Autodesk Fusion 360 part; units mm, degrees
(part 3 of 5)
sketch "スケッチ1 (2)" plane through (0, 0, 0) normal (0, 0, 1) x (1, 0, 0) in component "CasePlateExtended"
  spline S0 degree 3 poles (160.1864, -37.956) (159.9114, -37.956) (159.6865, -37.7311) (159.6865, -37.456) knots 0 0 0 0 1 1 1 1
  line L0 (159.6865, -37.456) -> (159.6865, -33.7563)
  spline S1 degree 3 poles (159.6865, -33.7563) (159.6865, -33.4812) (159.4615, -33.2562) (159.1863, -33.2562) knots 2 2 2 2 3 3 3 3
  line L1 (159.1863, -33.2562) -> (158.7622, -33.2562)
  spline S2 degree 3 poles (158.7622, -33.2562) (158.4869, -33.2562) (158.2619, -33.4812) (158.2619, -33.7563) knots 4 4 4 4 5 5 5 5
  line L2 (158.2619, -33.7563) -> (158.2619, -37.456)
  spline S3 degree 3 poles (158.2619, -37.456) (158.2619, -37.7311) (158.037, -37.956) (157.7621, -37.956) knots 6 6 6 6 7 7 7 7
  line L3 (157.7621, -37.956) -> (157.0372, -37.956)
  spline S4 degree 3 poles (157.0372, -37.956) (156.7619, -37.956) (156.537, -38.1743) (156.537, -38.7079) (156.312, -38.9262) (156.0371, -38.9262) knots 8 8 8 8 9 9 10 10 10 10
  line L4 (156.0371, -38.9262) -> (153.3871, -38.9262)
  spline S5 degree 3 poles (153.3871, -38.9262) (153.1119, -38.9262) (152.8869, -38.7079) (152.8869, -38.1743) (152.6619, -37.956) (152.387, -37.956) knots 11 11 11 11 12 12 13 13 13 13
  line L5 (152.387, -37.956) -> (143.5186, -37.956)
  spline S6 degree 3 poles (143.5186, -37.956) (143.2437, -37.956) (143.0188, -37.7311) (143.0188, -37.456) knots 14 14 14 14 15 15 15 15
  line L6 (143.0188, -37.456) -> (143.0188, -24.4562)
  spline S7 degree 3 poles (143.0188, -24.4562) (143.0188, -24.1811) (143.2437, -23.9562) (143.5186, -23.9562) knots 16 16 16 16 17 17 17 17
  line L7 (143.5186, -23.9562) -> (156.5184, -23.9562)
  spline S8 degree 3 poles (156.5184, -23.9562) (156.7936, -23.9562) (157.0186, -24.1744) (157.0186, -24.7077) (157.2436, -24.926) (157.5185, -24.926) knots 18 18 18 18 19 19 20 20 20 20
  line L8 (157.5185, -24.926) -> (157.7621, -24.926)
  spline S9 degree 3 poles (157.7621, -24.926) (158.037, -24.926) (158.2619, -25.1509) (158.2619, -25.426) knots 21 21 21 21 22 22 22 22
  line L9 (158.2619, -25.426) -> (158.2619, -28.1559)
  spline S10 degree 3 poles (158.2619, -28.1559) (158.2619, -28.431) (158.4869, -28.656) (158.7622, -28.656) knots 23 23 23 23 24 24 24 24
  line L10 (158.7622, -28.656) -> (159.1863, -28.656)
  spline S11 degree 3 poles (159.1863, -28.656) (159.4615, -28.656) (159.6865, -28.431) (159.6865, -28.1559) knots 25 25 25 25 26 26 26 26
  line L11 (159.6865, -28.1559) -> (159.6865, -24.4562)
  spline S12 degree 3 poles (159.6865, -24.4562) (159.6865, -24.1811) (159.9114, -23.9562) (160.1864, -23.9562) knots 27 27 27 27 28 28 28 28
  line L12 (160.1864, -23.9562) -> (182.7114, -23.9562)
  spline S13 degree 3 poles (182.7114, -23.9562) (182.9867, -23.9562) (183.2117, -24.1811) (183.2117, -24.4562) knots 29 29 29 29 30 30 30 30
  line L13 (183.2117, -24.4562) -> (183.2117, -37.456)
  spline S14 degree 3 poles (183.2117, -37.456) (183.2117, -37.7311) (182.9867, -37.956) (182.7114, -37.956) knots 31 31 31 31 32 32 32 32
  line L14 (182.7114, -37.956) -> (180.9861, -37.956)
  spline S15 degree 3 poles (180.9861, -37.956) (180.7109, -37.956) (180.4859, -38.1743) (180.4859, -38.7079) (180.261, -38.9262) (179.986, -38.9262) knots 33 33 33 33 34 34 35 35 35 35
  line L15 (179.986, -38.9262) -> (177.3371, -38.9262)
  spline S16 degree 3 poles (177.3371, -38.9262) (177.0618, -38.9262) (176.8369, -38.7079) (176.8369, -38.1743) (176.6119, -37.956) (176.337, -37.956) knots 36 36 36 36 37 37 38 38 38 38
  line L16 (176.337, -37.956) -> (160.1864, -37.956)
  spline S17 degree 3 poles (114.4437, -5.4062) (114.4437, -5.1311) (114.6687, -4.9062) (114.9436, -4.9062) knots 0 0 0 0 1 1 1 1
  line L17 (114.9436, -4.9062) -> (127.9434, -4.9062)
  spline S18 degree 3 poles (127.9434, -4.9062) (128.2186, -4.9062) (128.4436, -5.1311) (128.4436, -5.4062) knots 2 2 2 2 3 3 3 3
  line L18 (128.4436, -5.4062) -> (128.4436, -18.406)
  spline S19 degree 3 poles (128.4436, -18.406) (128.4436, -18.681) (128.2186, -18.906) (127.9434, -18.906) knots 4 4 4 4 5 5 5 5
  line L19 (127.9434, -18.906) -> (114.9436, -18.906)
  spline S20 degree 3 poles (114.9436, -18.906) (114.6687, -18.906) (114.4437, -18.681) (114.4437, -18.406) knots 6 6 6 6 7 7 7 7
  line L20 (114.4437, -18.406) -> (114.4437, -5.4062)
  spline S21 degree 3 poles (110.1804, 0.144) (109.9055, 0.144) (109.6805, 0.369) (109.6805, 0.6441) knots 0 0 0 0 1 1 1 1
  line L21 (109.6805, 0.6441) -> (109.6805, 13.6438)
  spline S22 degree 3 poles (109.6805, 13.6438) (109.6805, 13.9189) (109.9055, 14.1438) (110.1804, 14.1438) knots 2 2 2 2 3 3 3 3
  line L22 (110.1804, 14.1438) -> (123.1805, 14.1438)
  spline S23 degree 3 poles (123.1805, 14.1438) (123.4558, 14.1438) (123.6807, 13.9189) (123.6807, 13.6438) knots 4 4 4 4 5 5 5 5
  line L23 (123.6807, 13.6438) -> (123.6807, 0.6441)
  spline S24 degree 3 poles (123.6807, 0.6441) (123.6807, 0.369) (123.4558, 0.144) (123.1805, 0.144) knots 6 6 6 6 7 7 7 7
  line L24 (123.1805, 0.144) -> (110.1804, 0.144)
  line L25 (198.3818, 67.532) -> (-198.3818, 67.532)
  spline S25 degree 3 poles (-198.3818, 67.532) (-199.7568, 67.532) (-200.8816, 66.407) (-200.8816, 65.0321) knots 1 1 1 1 2 2 2 2
  line L26 (-200.8816, 65.0321) -> (-200.8816, -65.0319)
  spline S26 degree 3 poles (-200.8816, -65.0319) (-200.8816, -66.4072) (-199.7568, -67.532) (-198.3818, -67.532) knots 3 3 3 3 4 4 4 4
  line L27 (-198.3818, -67.532) -> (198.3818, -67.532)
  spline S27 degree 3 poles (198.3818, -67.532) (199.7564, -67.532) (200.8816, -66.4072) (200.8816, -65.0319) knots 5 5 5 5 6 6 6 6
  line L28 (200.8816, -65.0319) -> (200.8816, 65.0321)
  spline S28 degree 3 poles (200.8816, 65.0321) (200.8816, 66.407) (199.7564, 67.532) (198.3818, 67.532) knots 7 7 7 7 8 8 8 8
  spline S29 degree 3 poles (91.1304, 0.144) (90.8555, 0.144) (90.6305, 0.369) (90.6305, 0.6441) knots 0 0 0 0 1 1 1 1
  line L29 (90.6305, 0.6441) -> (90.6305, 13.6438)
  spline S30 degree 3 poles (90.6305, 13.6438) (90.6305, 13.9189) (90.8555, 14.1438) (91.1304, 14.1438) knots 2 2 2 2 3 3 3 3
  line L30 (91.1304, 14.1438) -> (104.1305, 14.1438)
  spline S31 degree 3 poles (104.1305, 14.1438) (104.4058, 14.1438) (104.6307, 13.9189) (104.6307, 13.6438) knots 4 4 4 4 5 5 5 5
  line L31 (104.6307, 13.6438) -> (104.6307, 0.6441)
  spline S32 degree 3 poles (104.6307, 0.6441) (104.6307, 0.369) (104.4058, 0.144) (104.1305, 0.144) knots 6 6 6 6 7 7 7 7
  line L32 (104.1305, 0.144) -> (91.1304, 0.144)
  spline S33 degree 3 poles (157.3056, 56.506) (157.3056, 56.7811) (157.5305, 57.006) (157.8055, 57.006) knots 0 0 0 0 1 1 1 1
  line L33 (157.8055, 57.006) -> (170.8055, 57.006)
  spline S34 degree 3 poles (170.8055, 57.006) (171.0808, 57.006) (171.3058, 56.7811) (171.3058, 56.506) knots 2 2 2 2 3 3 3 3
  line L34 (171.3058, 56.506) -> (171.3058, 43.5059)
  spline S35 degree 3 poles (171.3058, 43.5059) (171.3058, 43.2308) (171.0808, 43.0058) (170.8055, 43.0058) knots 4 4 4 4 5 5 5 5
  line L35 (170.8055, 43.0058) -> (157.8055, 43.0058)
  spline S36 degree 3 poles (157.8055, 43.0058) (157.5305, 43.0058) (157.3056, 43.2308) (157.3056, 43.5059) knots 6 6 6 6 7 7 7 7
  line L36 (157.3056, 43.5059) -> (157.3056, 56.506)
  spline S37 degree 3 poles (129.2304, 0.144) (128.9555, 0.144) (128.7306, 0.369) (128.7306, 0.6441) knots 0 0 0 0 1 1 1 1
  line L37 (128.7306, 0.6441) -> (128.7306, 13.6438)
  spline S38 degree 3 poles (128.7306, 13.6438) (128.7306, 13.9189) (128.9555, 14.1438) (129.2304, 14.1438) knots 2 2 2 2 3 3 3 3
  line L38 (129.2304, 14.1438) -> (142.2305, 14.1438)
  spline S39 degree 3 poles (142.2305, 14.1438) (142.5058, 14.1438) (142.7307, 13.9189) (142.7307, 13.6438) knots 4 4 4 4 5 5 5 5
  line L39 (142.7307, 13.6438) -> (142.7307, 0.6441)
  spline S40 degree 3 poles (142.7307, 0.6441) (142.7307, 0.369) (142.5058, 0.144) (142.2305, 0.144) knots 6 6 6 6 7 7 7 7
  line L40 (142.2305, 0.144) -> (129.2304, 0.144)
  spline S41 degree 3 poles (119.2056, 32.6938) (119.2056, 32.9689) (119.4305, 33.1939) (119.7054, 33.1939) knots 0 0 0 0 1 1 1 1
  line L41 (119.7054, 33.1939) -> (132.7055, 33.1939)
  spline S42 degree 3 poles (132.7055, 33.1939) (132.9808, 33.1939) (133.2057, 32.9689) (133.2057, 32.6938) knots 2 2 2 2 3 3 3 3
  line L42 (133.2057, 32.6938) -> (133.2057, 19.6941)
  spline S43 degree 3 poles (133.2057, 19.6941) (133.2057, 19.419) (132.9808, 19.194) (132.7055, 19.194) knots 4 4 4 4 5 5 5 5
  line L43 (132.7055, 19.194) -> (119.7054, 19.194)
  spline S44 degree 3 poles (119.7054, 19.194) (119.4305, 19.194) (119.2056, 19.419) (119.2056, 19.6941) knots 6 6 6 6 7 7 7 7
  line L44 (119.2056, 19.6941) -> (119.2056, 32.6938)
  spline S45 degree 3 poles (138.2556, 56.506) (138.2556, 56.7811) (138.4805, 57.006) (138.7554, 57.006) knots 0 0 0 0 1 1 1 1
  line L45 (138.7554, 57.006) -> (151.7555, 57.006)
  spline S46 degree 3 poles (151.7555, 57.006) (152.0308, 57.006) (152.2558, 56.7811) (152.2558, 56.506) knots 2 2 2 2 3 3 3 3
  line L46 (152.2558, 56.506) -> (152.2558, 43.5059)
  spline S47 degree 3 poles (152.2558, 43.5059) (152.2558, 43.2308) (152.0308, 43.0058) (151.7555, 43.0058) knots 4 4 4 4 5 5 5 5
  line L47 (151.7555, 43.0058) -> (138.7554, 43.0058)
  spline S48 degree 3 poles (138.7554, 43.0058) (138.4805, 43.0058) (138.2556, 43.2308) (138.2556, 43.5059) knots 6 6 6 6 7 7 7 7
  line L48 (138.2556, 43.5059) -> (138.2556, 56.506)
  spline S49 degree 3 poles (133.4937, -5.4062) (133.4937, -5.1311) (133.7187, -4.9062) (133.9936, -4.9062) knots 0 0 0 0 1 1 1 1
  line L49 (133.9936, -4.9062) -> (146.9934, -4.9062)
  spline S50 degree 3 poles (146.9934, -4.9062) (147.2686, -4.9062) (147.4936, -5.1311) (147.4936, -5.4062) knots 2 2 2 2 3 3 3 3
  line L50 (147.4936, -5.4062) -> (147.4936, -18.406)
  spline S51 degree 3 poles (147.4936, -18.406) (147.4936, -18.681) (147.2686, -18.906) (146.9934, -18.906) knots 4 4 4 4 5 5 5 5
  line L51 (146.9934, -18.906) -> (133.9936, -18.906)
  spline S52 degree 3 poles (133.9936, -18.906) (133.7187, -18.906) (133.4937, -18.681) (133.4937, -18.406) knots 6 6 6 6 7 7 7 7
  line L52 (133.4937, -18.406) -> (133.4937, -5.4062)
  spline S53 degree 3 poles (81.1055, 32.6938) (81.1055, 32.9689) (81.3305, 33.1939) (81.6054, 33.1939) knots 0 0 0 0 1 1 1 1
  line L53 (81.6054, 33.1939) -> (94.6055, 33.1939)
  spline S54 degree 3 poles (94.6055, 33.1939) (94.8807, 33.1939) (95.1057, 32.9689) (95.1057, 32.6938) knots 2 2 2 2 3 3 3 3
  line L54 (95.1057, 32.6938) -> (95.1057, 19.6941)
  spline S55 degree 3 poles (95.1057, 19.6941) (95.1057, 19.419) (94.8807, 19.194) (94.6055, 19.194) knots 4 4 4 4 5 5 5 5
  line L55 (94.6055, 19.194) -> (81.6054, 19.194)
  spline S56 degree 3 poles (81.6054, 19.194) (81.3305, 19.194) (81.1055, 19.419) (81.1055, 19.6941) knots 6 6 6 6 7 7 7 7
  line L56 (81.1055, 19.6941) -> (81.1055, 32.6938)
  spline S57 degree 3 poles (190.3558, 19.6941) (190.3558, 19.419) (190.1308, 19.194) (189.8555, 19.194) knots 0 0 0 0 1 1 1 1
  line L57 (189.8555, 19.194) -> (188.1302, 19.194)
  spline S58 degree 3 poles (188.1302, 19.194) (187.855, 19.194) (187.63, 18.9758) (187.63, 18.4421) (187.405, 18.2239) (187.1301, 18.2239) knots 2 2 2 2 3 3 4 4 4 4
  line L58 (187.1301, 18.2239) -> (184.4802, 18.2239)
  spline S59 degree 3 poles (184.4802, 18.2239) (184.2049, 18.2239) (183.9799, 18.4421) (183.9799, 18.9758) (183.755, 19.194) (183.48, 19.194) knots 5 5 5 5 6 6 7 7 7 7
  line L59 (183.48, 19.194) -> (164.1799, 19.194)
  spline S60 degree 3 poles (164.1799, 19.194) (163.905, 19.194) (163.68, 18.9758) (163.68, 18.4421) (163.4551, 18.2239) (163.1798, 18.2239) knots 8 8 8 8 9 9 10 10 10 10
  line L60 (163.1798, 18.2239) -> (160.5312, 18.2239)
  spline S61 degree 3 poles (160.5312, 18.2239) (160.256, 18.2239) (160.031, 18.4421) (160.031, 18.9758) (159.806, 19.194) (159.5311, 19.194) knots 11 11 11 11 12 12 13 13 13 13
  line L61 (159.5311, 19.194) -> (157.8055, 19.194)
  spline S62 degree 3 poles (157.8055, 19.194) (157.5305, 19.194) (157.3056, 19.419) (157.3056, 19.6941) knots 14 14 14 14 15 15 15 15
  line L62 (157.3056, 19.6941) -> (157.3056, 32.6938)
  spline S63 degree 3 poles (157.3056, 32.6938) (157.3056, 32.9689) (157.5305, 33.1939) (157.8055, 33.1939) knots 16 16 16 16 17 17 17 17
  line L63 (157.8055, 33.1939) -> (189.8555, 33.1939)
  spline S64 degree 3 poles (189.8555, 33.1939) (190.1308, 33.1939) (190.3558, 32.9689) (190.3558, 32.6938) knots 18 18 18 18 19 19 19 19
  line L64 (190.3558, 32.6938) -> (190.3558, 19.6941)
  line L65 (173.4745, 0.144) -> (172.0937, 0.144)
  spline S65 degree 3 poles (172.0937, 0.144) (171.8187, 0.144) (171.5938, 0.369) (171.5938, 0.6441) knots 1 1 1 1 2 2 2 2
  line L66 (171.5938, 0.6441) -> (171.5938, 13.6438)
  spline S66 degree 3 poles (171.5938, 13.6438) (171.5938, 13.9189) (171.8187, 14.1438) (172.0937, 14.1438) knots 3 3 3 3 4 4 4 4
  line L67 (172.0937, 14.1438) -> (185.0934, 14.1438)
  spline S67 degree 3 poles (185.0934, 14.1438) (185.3687, 14.1438) (185.5936, 13.9189) (185.5936, 13.369) (185.8186, 13.1441) (186.0935, 13.1441) knots 5 5 5 5 6 6 7 7 7 7
  line L68 (186.0935, 13.1441) -> (186.5038, 13.1441)
  spline S68 degree 3 poles (186.5038, 13.1441) (186.7791, 13.1441) (187.004, 12.9191) (187.004, 12.644) knots 8 8 8 8 9 9 9 9
  line L69 (187.004, 12.644) -> (187.004, 6.5441)
  spline S69 degree 3 poles (187.004, 6.5441) (187.004, 6.269) (186.7791, 6.0441) (186.5038, 6.0441) knots 10 10 10 10 11 11 11 11
  line L70 (186.5038, 6.0441) -> (186.0935, 6.0441)
  spline S70 degree 3 poles (186.0935, 6.0441) (185.8186, 6.0441) (185.5936, 5.8191) (185.5936, 5.544) knots 12 12 12 12 13 13 13 13
  line L71 (185.5936, 5.544) -> (185.5936, 5.1189)
  spline S71 degree 3 poles (185.5936, 5.1189) (185.5936, 4.8438) (185.8186, 4.6188) (186.0935, 4.6188) knots 14 14 14 14 15 15 15 15
  line L72 (186.0935, 4.6188) -> (187.4743, 4.6188)
  spline S72 degree 3 poles (187.4743, 4.6188) (187.7496, 4.6188) (187.9745, 4.3939) (187.9745, 4.1188) knots 16 16 16 16 17 17 17 17
  line L73 (187.9745, 4.1188) -> (187.9745, -8.8809)
  spline S73 degree 3 poles (187.9745, -8.8809) (187.9745, -9.156) (187.7561, -9.381) (187.4891, -9.381) (187.2225, -9.381) (187.004, -9.606) (187.004, -9.8811) knots 18 18 18 18 19 19 19 20 20 20 20
  line L74 (187.004, -9.8811) -> (187.004, -10.9063)
  spline S74 degree 3 poles (187.004, -10.9063) (187.004, -11.1814) (187.1267, -11.4064) (187.2769, -11.4064) (187.4268, -11.4064) (187.5497, -11.6313) (187.5497, -11.9064) knots 21 21 21 21 22 22 22 23 23 23 23
  line L75 (187.5497, -11.9064) -> (187.5497, -13.7065)
  spline S75 degree 3 poles (187.5497, -13.7065) (187.5497, -13.9816) (187.4268, -14.2065) (187.2769, -14.2065) (187.1267, -14.2065) (187.004, -14.4315) (187.004, -14.7066) knots 24 24 24 24 25 25 25 26 26 26 26
  line L76 (187.004, -14.7066) -> (187.004, -17.436)
  spline S76 degree 3 poles (187.004, -17.436) (187.004, -17.7111) (186.7791, -17.936) (186.5038, -17.936) knots 27 27 27 27 28 28 28 28
  line L77 (186.5038, -17.936) -> (183.7746, -17.936)
  spline S77 degree 3 poles (183.7746, -17.936) (183.4997, -17.936) (183.2747, -18.0587) (183.2747, -18.2087) (183.2747, -18.3586) (183.0498, -18.4812) (182.7745, -18.4812) knots 29 29 29 29 30 30 30 31 31 31 31
  line L78 (182.7745, -18.4812) -> (180.9744, -18.4812)
  spline S78 degree 3 poles (180.9744, -18.4812) (180.6995, -18.4812) (180.4745, -18.3586) (180.4745, -18.2087) (180.4745, -18.0587) (180.2496, -17.936) (179.9743, -17.936) knots 32 32 32 32 33 33 33 34 34 34 34
  line L79 (179.9743, -17.936) -> (178.9494, -17.936)
  spline S79 degree 3 poles (178.9494, -17.936) (178.6745, -17.936) (178.4495, -18.1543) (178.4495, -18.4213) (178.4495, -18.6881) (178.2246, -18.9064) (177.9493, -18.9064) knots 35 35 35 35 36 36 36 37 37 37 37
  line L80 (177.9493, -18.9064) -> (153.0436, -18.906)
  spline S80 degree 3 poles (153.0436, -18.906) (152.7687, -18.906) (152.5438, -18.681) (152.5438, -18.406) knots 38 38 38 38 39 39 39 39
  line L81 (152.5438, -18.406) -> (152.5438, -5.4062)
  spline S81 degree 3 poles (152.5438, -5.4062) (152.5438, -5.1311) (152.7687, -4.9062) (153.0436, -4.9062) knots 40 40 40 40 41 41 41 41
  line L82 (153.0436, -4.9062) -> (157.1488, -4.9062)
  spline S82 degree 3 poles (157.1488, -4.9062) (157.4241, -4.9062) (157.6491, -4.6879) (157.6491, -4.1546) (157.874, -3.9364) (158.1489, -3.9364) knots 42 42 42 42 43 43 44 44 44 44
  line L83 (158.1489, -3.9364) -> (160.7989, -3.9364)
  spline S83 degree 3 poles (160.7989, -3.9364) (161.0742, -3.9364) (161.2991, -4.1546) (161.2991, -4.6879) (161.5241, -4.9062) (161.799, -4.9062) knots 45 45 45 45 46 46 47 47 47 47
  line L84 (161.799, -4.9062) -> (173.4745, -4.9065)
  spline S84 degree 3 poles (173.4745, -4.9065) (173.7497, -4.9065) (173.9747, -4.6815) (173.9747, -4.4065) knots 48 48 48 48 49 49 49 49
  line L85 (173.9747, -4.4065) -> (173.9747, -0.3561)
  spline S85 degree 3 poles (173.9747, -0.3561) (173.9747, -0.081) (173.7497, 0.144) (173.4745, 0.144) knots 50 50 50 50 51 51 51 51
  spline S86 degree 3 poles (100.1555, 56.506) (100.1555, 56.7811) (100.3805, 57.006) (100.6554, 57.006) knots 0 0 0 0 1 1 1 1
  line L86 (100.6554, 57.006) -> (113.6555, 57.006)
  spline S87 degree 3 poles (113.6555, 57.006) (113.9308, 57.006) (114.1557, 56.7811) (114.1557, 56.506) knots 2 2 2 2 3 3 3 3
  line L87 (114.1557, 56.506) -> (114.1557, 43.5059)
  spline S88 degree 3 poles (114.1557, 43.5059) (114.1557, 43.2308) (113.9308, 43.0058) (113.6555, 43.0058) knots 4 4 4 4 5 5 5 5
  line L88 (113.6555, 43.0058) -> (100.6554, 43.0058)
  spline S89 degree 3 poles (100.6554, 43.0058) (100.3805, 43.0058) (100.1555, 43.2308) (100.1555, 43.5059) knots 6 6 6 6 7 7 7 7
  line L89 (100.1555, 43.5059) -> (100.1555, 56.506)
  spline S90 degree 3 poles (190.3558, 43.5059) (190.3558, 43.2308) (190.1308, 43.0058) (189.8555, 43.0058) knots 0 0 0 0 1 1 1 1
  line L90 (189.8555, 43.0058) -> (176.8555, 43.0058)
  spline S91 degree 3 poles (176.8555, 43.0058) (176.5806, 43.0058) (176.3556, 43.2308) (176.3556, 43.5059) knots 2 2 2 2 3 3 3 3
  line L91 (176.3556, 43.5059) -> (176.3556, 56.506)
  spline S92 degree 3 poles (176.3556, 56.506) (176.3556, 56.7811) (176.5806, 57.006) (176.8555, 57.006) knots 4 4 4 4 5 5 5 5
  line L92 (176.8555, 57.006) -> (189.8555, 57.006)
  spline S93 degree 3 poles (189.8555, 57.006) (190.1308, 57.006) (190.3558, 56.7811) (190.3558, 56.506) knots 6 6 6 6 7 7 7 7
  line L93 (190.3558, 56.506) -> (190.3558, 43.5059)
  spline S94 degree 3 poles (138.2556, 32.6938) (138.2556, 32.9689) (138.4805, 33.1939) (138.7554, 33.1939) knots 0 0 0 0 1 1 1 1
  line L94 (138.7554, 33.1939) -> (151.7555, 33.1939)
  spline S95 degree 3 poles (151.7555, 33.1939) (152.0308, 33.1939) (152.2558, 32.9689) (152.2558, 32.6938) knots 2 2 2 2 3 3 3 3
  line L95 (152.2558, 32.6938) -> (152.2558, 19.6941)
  spline S96 degree 3 poles (152.2558, 19.6941) (152.2558, 19.419) (152.0308, 19.194) (151.7555, 19.194) knots 4 4 4 4 5 5 5 5
  line L96 (151.7555, 19.194) -> (138.7554, 19.194)
  spline S97 degree 3 poles (138.7554, 19.194) (138.4805, 19.194) (138.2556, 19.419) (138.2556, 19.6941) knots 6 6 6 6 7 7 7 7
  line L97 (138.2556, 19.6941) -> (138.2556, 32.6938)
  spline S98 degree 3 poles (161.7808, 0.6441) (161.7808, 0.369) (161.5558, 0.144) (161.2805, 0.144) knots 0 0 0 0 1 1 1 1
  line L98 (161.2805, 0.144) -> (148.2805, 0.144)
  spline S99 degree 3 poles (148.2805, 0.144) (148.0055, 0.144) (147.7806, 0.369) (147.7806, 0.6441) knots 2 2 2 2 3 3 3 3
  line L99 (147.7806, 0.6441) -> (147.7806, 13.6438)
  spline S100 degree 3 poles (147.7806, 13.6438) (147.7806, 13.9189) (148.0055, 14.1438) (148.2805, 14.1438) knots 4 4 4 4 5 5 5 5
  line L100 (148.2805, 14.1438) -> (161.2805, 14.1438)
  spline S101 degree 3 poles (161.2805, 14.1438) (161.5558, 14.1438) (161.7808, 13.9189) (161.7808, 13.6438) knots 6 6 6 6 7 7 7 7
  line L101 (161.7808, 13.6438) -> (161.7808, 0.6441)
  spline S102 degree 3 poles (119.2056, 56.506) (119.2056, 56.7811) (119.4305, 57.006) (119.7054, 57.006) knots 0 0 0 0 1 1 1 1
  line L102 (119.7054, 57.006) -> (132.7055, 57.006)
  spline S103 degree 3 poles (132.7055, 57.006) (132.9808, 57.006) (133.2057, 56.7811) (133.2057, 56.506) knots 2 2 2 2 3 3 3 3
  line L103 (133.2057, 56.506) -> (133.2057, 43.5059)
  spline S104 degree 3 poles (133.2057, 43.5059) (133.2057, 43.2308) (132.9808, 43.0058) (132.7055, 43.0058) knots 4 4 4 4 5 5 5 5
  line L104 (132.7055, 43.0058) -> (119.7054, 43.0058)
  spline S105 degree 3 poles (119.7054, 43.0058) (119.4305, 43.0058) (119.2056, 43.2308) (119.2056, 43.5059) knots 6 6 6 6 7 7 7 7
  line L105 (119.2056, 43.5059) -> (119.2056, 56.506)
  spline S106 degree 3 poles (100.1555, 32.6938) (100.1555, 32.9689) (100.3805, 33.1939) (100.6554, 33.1939) knots 0 0 0 0 1 1 1 1
  line L106 (100.6554, 33.1939) -> (113.6555, 33.1939)
  spline S107 degree 3 poles (113.6555, 33.1939) (113.9308, 33.1939) (114.1557, 32.9689) (114.1557, 32.6938) knots 2 2 2 2 3 3 3 3
  line L107 (114.1557, 32.6938) -> (114.1557, 19.6941)
  spline S108 degree 3 poles (114.1557, 19.6941) (114.1557, 19.419) (113.9308, 19.194) (113.6555, 19.194) knots 4 4 4 4 5 5 5 5
  line L108 (113.6555, 19.194) -> (100.6554, 19.194)
  spline S109 degree 3 poles (100.6554, 19.194) (100.3805, 19.194) (100.1555, 19.419) (100.1555, 19.6941) knots 6 6 6 6 7 7 7 7
  line L109 (100.1555, 19.6941) -> (100.1555, 32.6938)
  spline S110 degree 3 poles (190.3558, -56.506) (190.3558, -56.7811) (190.1308, -57.006) (189.8555, -57.006) knots 0 0 0 0 1 1 1 1
  line L110 (189.8555, -57.006) -> (176.8555, -57.006)
  spline S111 degree 3 poles (176.8555, -57.006) (176.5806, -57.006) (176.3556, -56.7811) (176.3556, -56.506) knots 2 2 2 2 3 3 3 3
  line L111 (176.3556, -56.506) -> (176.3556, -43.5062)
  spline S112 degree 3 poles (176.3556, -43.5062) (176.3556, -43.2312) (176.5806, -43.0062) (176.8555, -43.0062) knots 4 4 4 4 5 5 5 5
  line L112 (176.8555, -43.0062) -> (189.8555, -43.0062)
  spline S113 degree 3 poles (189.8555, -43.0062) (190.1308, -43.0062) (190.3558, -43.2312) (190.3558, -43.5062) knots 6 6 6 6 7 7 7 7
  line L113 (190.3558, -43.5062) -> (190.3558, -56.506)
  spline S114 degree 3 poles (-138.2566, 24.4559) (-138.2566, 24.1808) (-138.4816, 23.9558) (-138.7568, 23.9558) knots 0 0 0 0 1 1 1 1
  line L114 (-138.7568, 23.9558) -> (-151.7569, 23.9558)
  spline S115 degree 3 poles (-151.7569, 23.9558) (-152.0318, 23.9558) (-152.2568, 24.1808) (-152.2568, 24.4559) knots 2 2 2 2 3 3 3 3
  line L115 (-152.2568, 24.4559) -> (-152.2568, 37.456)
  spline S116 degree 3 poles (-152.2568, 37.456) (-152.2568, 37.7311) (-152.0318, 37.956) (-151.7569, 37.956) knots 4 4 4 4 5 5 5 5
  line L116 (-151.7569, 37.956) -> (-138.7568, 37.956)
  spline S117 degree 3 poles (-138.7568, 37.956) (-138.4816, 37.956) (-138.2566, 37.7311) (-138.2566, 37.456) knots 6 6 6 6 7 7 7 7
  line L117 (-138.2566, 37.456) -> (-138.2566, 24.4559)
  spline S118 degree 3 poles (19.6936, -18.906) (19.4186, -18.906) (19.1937, -18.681) (19.1937, -18.406) knots 0 0 0 0 1 1 1 1
  line L118 (19.1937, -18.406) -> (19.1937, -5.4062)
  spline S119 degree 3 poles (19.1937, -5.4062) (19.1937, -5.1311) (19.4186, -4.9062) (19.6936, -4.9062) knots 2 2 2 2 3 3 3 3
  line L119 (19.6936, -4.9062) -> (32.6933, -4.9062)
  spline S120 degree 3 poles (32.6933, -4.9062) (32.9686, -4.9062) (33.1935, -5.1311) (33.1935, -5.4062) knots 4 4 4 4 5 5 5 5
  line L120 (33.1935, -5.4062) -> (33.1935, -18.406)
  spline S121 degree 3 poles (33.1935, -18.406) (33.1935, -18.681) (32.9686, -18.906) (32.6933, -18.906) knots 6 6 6 6 7 7 7 7
  line L121 (32.6933, -18.906) -> (19.6936, -18.906)
  spline S122 degree 3 poles (-90.3446, 56.506) (-90.3446, 56.7811) (-90.1196, 57.006) (-89.8447, 57.006) knots 0 0 0 0 1 1 1 1
  line L122 (-89.8447, 57.006) -> (-76.845, 57.006)
  spline S123 degree 3 poles (-76.845, 57.006) (-76.5697, 57.006) (-76.3447, 56.7811) (-76.3447, 56.506) knots 2 2 2 2 3 3 3 3
  line L123 (-76.3447, 56.506) -> (-76.3447, 43.5059)
  spline S124 degree 3 poles (-76.3447, 43.5059) (-76.3447, 43.2308) (-76.5697, 43.0058) (-76.845, 43.0058) knots 4 4 4 4 5 5 5 5
  line L124 (-76.845, 43.0058) -> (-89.8447, 43.0058)
  spline S125 degree 3 poles (-89.8447, 43.0058) (-90.1196, 43.0058) (-90.3446, 43.2308) (-90.3446, 43.5059) knots 6 6 6 6 7 7 7 7
  line L125 (-90.3446, 43.5059) -> (-90.3446, 56.506)
  spline S126 degree 3 poles (-37.9564, -5.4062) (-37.9564, -5.1311) (-37.7314, -4.9062) (-37.4565, -4.9062) knots 0 0 0 0 1 1 1 1
  line L126 (-37.4565, -4.9062) -> (-24.4567, -4.9062)
  spline S127 degree 3 poles (-24.4567, -4.9062) (-24.1815, -4.9062) (-23.9565, -5.1311) (-23.9565, -5.4062) knots 2 2 2 2 3 3 3 3
  line L127 (-23.9565, -5.4062) -> (-23.9565, -18.406)
  spline S128 degree 3 poles (-23.9565, -18.406) (-23.9565, -18.681) (-24.1815, -18.906) (-24.4567, -18.906) knots 4 4 4 4 5 5 5 5
  line L128 (-24.4567, -18.906) -> (-37.4565, -18.906)
  spline S129 degree 3 poles (-37.4565, -18.906) (-37.7314, -18.906) (-37.9564, -18.681) (-37.9564, -18.406) knots 6 6 6 6 7 7 7 7
  line L129 (-37.9564, -18.406) -> (-37.9564, -5.4062)
  line L130 (14.4305, 0.6441) -> (14.4305, 13.6438)
  spline S130 degree 3 poles (14.4305, 13.6438) (14.4305, 13.9189) (14.6554, 14.1438) (14.9304, 14.1438) knots 1 1 1 1 2 2 2 2
  line L131 (14.9304, 14.1438) -> (27.9304, 14.1438)
  spline S131 degree 3 poles (27.9304, 14.1438) (28.2057, 14.1438) (28.4307, 13.9189) (28.4307, 13.6438) knots 3 3 3 3 4 4 4 4
  line L132 (28.4307, 13.6438) -> (28.4307, 0.6441)
  spline S132 degree 3 poles (28.4307, 0.6441) (28.4307, 0.369) (28.2057, 0.144) (27.9304, 0.144) knots 5 5 5 5 6 6 6 6
  line L133 (27.9304, 0.144) -> (14.9304, 0.144)
  spline S133 degree 3 poles (14.9304, 0.144) (14.6554, 0.144) (14.4305, 0.369) (14.4305, 0.6441) knots 7 7 7 7 8 8 8 8
  spline S134 degree 3 poles (9.6687, -24.4562) (9.6687, -24.1811) (9.8936, -23.9562) (10.1686, -23.9562) knots 0 0 0 0 1 1 1 1
  line L134 (10.1686, -23.9562) -> (23.1683, -23.9562)
  spline S135 degree 3 poles (23.1683, -23.9562) (23.4435, -23.9562) (23.6685, -24.1811) (23.6685, -24.4562) knots 2 2 2 2 3 3 3 3
  line L135 (23.6685, -24.4562) -> (23.6685, -37.456)
  spline S136 degree 3 poles (23.6685, -37.456) (23.6685, -37.7311) (23.4435, -37.956) (23.1683, -37.956) knots 4 4 4 4 5 5 5 5
  line L136 (23.1683, -37.956) -> (10.1686, -37.956)
  spline S137 degree 3 poles (10.1686, -37.956) (9.8936, -37.956) (9.6687, -37.7311) (9.6687, -37.456) knots 6 6 6 6 7 7 7 7
  line L137 (9.6687, -37.456) -> (9.6687, -24.4562)
  line L138 (71.5805, 0.6441) -> (71.5805, 13.6438)
  spline S138 degree 3 poles (71.5805, 13.6438) (71.5805, 13.9189) (71.8055, 14.1438) (72.0804, 14.1438) knots 1 1 1 1 2 2 2 2
  line L139 (72.0804, 14.1438) -> (85.0805, 14.1438)
  spline S139 degree 3 poles (85.0805, 14.1438) (85.3557, 14.1438) (85.5807, 13.9189) (85.5807, 13.6438) knots 3 3 3 3 4 4 4 4
  line L140 (85.5807, 13.6438) -> (85.5807, 0.6441)
  spline S140 degree 3 poles (85.5807, 0.6441) (85.5807, 0.369) (85.3557, 0.144) (85.0805, 0.144) knots 5 5 5 5 6 6 6 6
  line L141 (85.0805, 0.144) -> (72.0804, 0.144)
  spline S141 degree 3 poles (72.0804, 0.144) (71.8055, 0.144) (71.5805, 0.369) (71.5805, 0.6441) knots 7 7 7 7 8 8 8 8
  spline S142 degree 3 poles (66.8187, -24.4562) (66.8187, -24.1811) (67.0437, -23.9562) (67.3186, -23.9562) knots 0 0 0 0 1 1 1 1
  line L142 (67.3186, -23.9562) -> (80.3183, -23.9562)
  spline S143 degree 3 poles (80.3183, -23.9562) (80.5936, -23.9562) (80.8185, -24.1811) (80.8185, -24.4562) knots 2 2 2 2 3 3 3 3
  line L143 (80.8185, -24.4562) -> (80.8185, -37.456)
  spline S144 degree 3 poles (80.8185, -37.456) (80.8185, -37.7311) (80.5936, -37.956) (80.3183, -37.956) knots 4 4 4 4 5 5 5 5
  line L144 (80.3183, -37.956) -> (67.3186, -37.956)
  spline S145 degree 3 poles (67.3186, -37.956) (67.0437, -37.956) (66.8187, -37.7311) (66.8187, -37.456) knots 6 6 6 6 7 7 7 7
  line L145 (66.8187, -37.456) -> (66.8187, -24.4562)
  spline S146 degree 3 poles (-9.3813, -24.4562) (-9.3813, -24.1811) (-9.1564, -23.9562) (-8.8815, -23.9562) knots 0 0 0 0 1 1 1 1
  line L146 (-8.8815, -23.9562) -> (4.1183, -23.9562)
  spline S147 degree 3 poles (4.1183, -23.9562) (4.3935, -23.9562) (4.6185, -24.1811) (4.6185, -24.4562) knots 2 2 2 2 3 3 3 3
  line L147 (4.6185, -24.4562) -> (4.6185, -37.456)
  spline S148 degree 3 poles (4.6185, -37.456) (4.6185, -37.7311) (4.3935, -37.956) (4.1183, -37.956) knots 4 4 4 4 5 5 5 5
  line L148 (4.1183, -37.956) -> (-8.8815, -37.956)
  spline S149 degree 3 poles (-8.8815, -37.956) (-9.1564, -37.956) (-9.3813, -37.7311) (-9.3813, -37.456) knots 6 6 6 6 7 7 7 7
  line L149 (-9.3813, -37.456) -> (-9.3813, -24.4562)
  spline S150 degree 3 poles (62.0555, 56.506) (62.0555, 56.7811) (62.2805, 57.006) (62.5554, 57.006) knots 0 0 0 0 1 1 1 1
  line L150 (62.5554, 57.006) -> (75.5555, 57.006)
  spline S151 degree 3 poles (75.5555, 57.006) (75.8307, 57.006) (76.0557, 56.7811) (76.0557, 56.506) knots 2 2 2 2 3 3 3 3
  line L151 (76.0557, 56.506) -> (76.0557, 43.5059)
  spline S152 degree 3 poles (76.0557, 43.5059) (76.0557, 43.2308) (75.8307, 43.0058) (75.5555, 43.0058) knots 4 4 4 4 5 5 5 5
  line L152 (75.5555, 43.0058) -> (62.5554, 43.0058)
  spline S153 degree 3 poles (62.5554, 43.0058) (62.2805, 43.0058) (62.0555, 43.2308) (62.0555, 43.5059) knots 6 6 6 6 7 7 7 7
  line L153 (62.0555, 43.5059) -> (62.0555, 56.506)
  spline S154 degree 3 poles (81.1055, 56.506) (81.1055, 56.7811) (81.3305, 57.006) (81.6054, 57.006) knots 0 0 0 0 1 1 1 1
  line L154 (81.6054, 57.006) -> (94.6055, 57.006)
  spline S155 degree 3 poles (94.6055, 57.006) (94.8807, 57.006) (95.1057, 56.7811) (95.1057, 56.506) knots 2 2 2 2 3 3 3 3
  line L155 (95.1057, 56.506) -> (95.1057, 43.5059)
  spline S156 degree 3 poles (95.1057, 43.5059) (95.1057, 43.2308) (94.8807, 43.0058) (94.6055, 43.0058) knots 4 4 4 4 5 5 5 5
  line L156 (94.6055, 43.0058) -> (81.6054, 43.0058)
  spline S157 degree 3 poles (81.6054, 43.0058) (81.3305, 43.0058) (81.1055, 43.2308) (81.1055, 43.5059) knots 6 6 6 6 7 7 7 7
  line L157 (81.1055, 43.5059) -> (81.1055, 56.506)
  spline S158 degree 3 poles (0.6435, -18.906) (0.3686, -18.906) (0.1437, -18.681) (0.1437, -18.406) knots 0 0 0 0 1 1 1 1
  line L158 (0.1437, -18.406) -> (0.1437, -5.4062)
  spline S159 degree 3 poles (0.1437, -5.4062) (0.1437, -5.1311) (0.3686, -4.9062) (0.6435, -4.9062) knots 2 2 2 2 3 3 3 3
  line L159 (0.6435, -4.9062) -> (13.6433, -4.9062)
  spline S160 degree 3 poles (13.6433, -4.9062) (13.9185, -4.9062) (14.1435, -5.1311) (14.1435, -5.4062) knots 4 4 4 4 5 5 5 5
  line L160 (14.1435, -5.4062) -> (14.1435, -18.406)
  spline S161 degree 3 poles (14.1435, -18.406) (14.1435, -18.681) (13.9185, -18.906) (13.6433, -18.906) knots 6 6 6 6 7 7 7 7
  line L161 (13.6433, -18.906) -> (0.6435, -18.906)
  line L162 (52.5305, 0.6441) -> (52.5305, 13.6438)
  spline S162 degree 3 poles (52.5305, 13.6438) (52.5305, 13.9189) (52.7555, 14.1438) (53.0304, 14.1438) knots 1 1 1 1 2 2 2 2
  line L163 (53.0304, 14.1438) -> (66.0305, 14.1438)
  spline S163 degree 3 poles (66.0305, 14.1438) (66.3057, 14.1438) (66.5307, 13.9189) (66.5307, 13.6438) knots 3 3 3 3 4 4 4 4
  line L164 (66.5307, 13.6438) -> (66.5307, 0.6441)
  spline S164 degree 3 poles (66.5307, 0.6441) (66.5307, 0.369) (66.3057, 0.144) (66.0305, 0.144) knots 5 5 5 5 6 6 6 6
  line L165 (66.0305, 0.144) -> (53.0304, 0.144)
  spline S165 degree 3 poles (53.0304, 0.144) (52.7555, 0.144) (52.5305, 0.369) (52.5305, 0.6441) knots 7 7 7 7 8 8 8 8
  spline S166 degree 3 poles (62.0555, 32.6938) (62.0555, 32.9689) (62.2805, 33.1939) (62.5554, 33.1939) knots 0 0 0 0 1 1 1 1
  line L166 (62.5554, 33.1939) -> (75.5555, 33.1939)
  spline S167 degree 3 poles (75.5555, 33.1939) (75.8307, 33.1939) (76.0557, 32.9689) (76.0557, 32.6938) knots 2 2 2 2 3 3 3 3
  line L167 (76.0557, 32.6938) -> (76.0557, 19.6941)
  spline S168 degree 3 poles (76.0557, 19.6941) (76.0557, 19.419) (75.8307, 19.194) (75.5555, 19.194) knots 4 4 4 4 5 5 5 5
  line L168 (75.5555, 19.194) -> (62.5554, 19.194)
  spline S169 degree 3 poles (62.5554, 19.194) (62.2805, 19.194) (62.0555, 19.419) (62.0555, 19.6941) knots 6 6 6 6 7 7 7 7
  line L169 (62.0555, 19.6941) -> (62.0555, 32.6938)
  spline S170 degree 3 poles (23.9555, 32.6938) (23.9555, 32.9689) (24.1805, 33.1939) (24.4554, 33.1939) knots 0 0 0 0 1 1 1 1
  line L170 (24.4554, 33.1939) -> (37.4554, 33.1939)
  spline S171 degree 3 poles (37.4554, 33.1939) (37.7307, 33.1939) (37.9557, 32.9689) (37.9557, 32.6938) knots 2 2 2 2 3 3 3 3
  line L171 (37.9557, 32.6938) -> (37.9557, 19.6941)
  spline S172 degree 3 poles (37.9557, 19.6941) (37.9557, 19.419) (37.7307, 19.194) (37.4554, 19.194) knots 4 4 4 4 5 5 5 5
  line L172 (37.4554, 19.194) -> (24.4554, 19.194)
  spline S173 degree 3 poles (24.4554, 19.194) (24.1805, 19.194) (23.9555, 19.419) (23.9555, 19.6941) knots 6 6 6 6 7 7 7 7
  line L173 (23.9555, 19.6941) -> (23.9555, 32.6938)
  spline S174 degree 3 poles (-42.2197, 0.144) (-42.4946, 0.144) (-42.7196, 0.369) (-42.7196, 0.6441) knots 0 0 0 0 1 1 1 1
  line L174 (-42.7196, 0.6441) -> (-42.7196, 13.6438)
  spline S175 degree 3 poles (-42.7196, 13.6438) (-42.7196, 13.9189) (-42.4946, 14.1438) (-42.2197, 14.1438) knots 2 2 2 2 3 3 3 3
  line L175 (-42.2197, 14.1438) -> (-29.2196, 14.1438)
  spline S176 degree 3 poles (-29.2196, 14.1438) (-28.9443, 14.1438) (-28.7194, 13.9189) (-28.7194, 13.6438) knots 4 4 4 4 5 5 5 5
  line L176 (-28.7194, 13.6438) -> (-28.7194, 0.6441)
  spline S177 degree 3 poles (-28.7194, 0.6441) (-28.7194, 0.369) (-28.9443, 0.144) (-29.2196, 0.144) knots 6 6 6 6 7 7 7 7
  line L177 (-29.2196, 0.144) -> (-42.2197, 0.144)
  spline S178 degree 3 poles (-52.2446, 32.6938) (-52.2446, 32.9689) (-52.0196, 33.1939) (-51.7447, 33.1939) knots 0 0 0 0 1 1 1 1
  line L178 (-51.7447, 33.1939) -> (-38.7446, 33.1939)
  spline S179 degree 3 poles (-38.7446, 33.1939) (-38.4693, 33.1939) (-38.2444, 32.9689) (-38.2444, 32.6938) knots 2 2 2 2 3 3 3 3
  line L179 (-38.2444, 32.6938) -> (-38.2444, 19.6941)
  spline S180 degree 3 poles (-38.2444, 19.6941) (-38.2444, 19.419) (-38.4693, 19.194) (-38.7446, 19.194) knots 4 4 4 4 5 5 5 5
  line L180 (-38.7446, 19.194) -> (-51.7447, 19.194)
  spline S181 degree 3 poles (-51.7447, 19.194) (-52.0196, 19.194) (-52.2446, 19.419) (-52.2446, 19.6941) knots 6 6 6 6 7 7 7 7
  line L181 (-52.2446, 19.6941) -> (-52.2446, 32.6938)
  spline S182 degree 3 poles (-61.2697, 0.144) (-61.5446, 0.144) (-61.7696, 0.369) (-61.7696, 0.6441) knots 0 0 0 0 1 1 1 1
  line L182 (-61.7696, 0.6441) -> (-61.7696, 13.6438)
  spline S183 degree 3 poles (-61.7696, 13.6438) (-61.7696, 13.9189) (-61.5446, 14.1438) (-61.2697, 14.1438) knots 2 2 2 2 3 3 3 3
  line L183 (-61.2697, 14.1438) -> (-48.2696, 14.1438)
  spline S184 degree 3 poles (-48.2696, 14.1438) (-47.9943, 14.1438) (-47.7694, 13.9189) (-47.7694, 13.6438) knots 4 4 4 4 5 5 5 5
  line L184 (-47.7694, 13.6438) -> (-47.7694, 0.6441)
  spline S185 degree 3 poles (-47.7694, 0.6441) (-47.7694, 0.369) (-47.9943, 0.144) (-48.2696, 0.144) knots 6 6 6 6 7 7 7 7
  line L185 (-48.2696, 0.144) -> (-61.2697, 0.144)
  spline S186 degree 3 poles (-71.2946, 32.6938) (-71.2946, 32.9689) (-71.0696, 33.1939) (-70.7947, 33.1939) knots 0 0 0 0 1 1 1 1
  line L186 (-70.7947, 33.1939) -> (-57.795, 33.1939)
  spline S187 degree 3 poles (-57.795, 33.1939) (-57.5197, 33.1939) (-57.2947, 32.9689) (-57.2947, 32.6938) knots 2 2 2 2 3 3 3 3
  line L187 (-57.2947, 32.6938) -> (-57.2947, 19.6941)
  spline S188 degree 3 poles (-57.2947, 19.6941) (-57.2947, 19.419) (-57.5197, 19.194) (-57.795, 19.194) knots 4 4 4 4 5 5 5 5
  line L188 (-57.795, 19.194) -> (-70.7947, 19.194)
  spline S189 degree 3 poles (-70.7947, 19.194) (-71.0696, 19.194) (-71.2946, 19.419) (-71.2946, 19.6941) knots 6 6 6 6 7 7 7 7
  line L189 (-71.2946, 19.6941) -> (-71.2946, 32.6938)
  spline S190 degree 3 poles (-90.3446, 32.6938) (-90.3446, 32.9689) (-90.1196, 33.1939) (-89.8447, 33.1939) knots 0 0 0 0 1 1 1 1
  line L190 (-89.8447, 33.1939) -> (-76.845, 33.1939)
  spline S191 degree 3 poles (-76.845, 33.1939) (-76.5697, 33.1939) (-76.3447, 32.9689) (-76.3447, 32.6938) knots 2 2 2 2 3 3 3 3
  line L191 (-76.3447, 32.6938) -> (-76.3447, 19.6941)
  spline S192 degree 3 poles (-76.3447, 19.6941) (-76.3447, 19.419) (-76.5697, 19.194) (-76.845, 19.194) knots 4 4 4 4 5 5 5 5
  line L192 (-76.845, 19.194) -> (-89.8447, 19.194)
  spline S193 degree 3 poles (-89.8447, 19.194) (-90.1196, 19.194) (-90.3446, 19.419) (-90.3446, 19.6941) knots 6 6 6 6 7 7 7 7
  line L193 (-90.3446, 19.6941) -> (-90.3446, 32.6938)
  spline S194 degree 3 poles (-176.3566, -18.406) (-176.3566, -18.681) (-176.5816, -18.906) (-176.8568, -18.906) knots 0 0 0 0 1 1 1 1
  line L194 (-176.8568, -18.906) -> (-189.8569, -18.906)
  spline S195 degree 3 poles (-189.8569, -18.906) (-190.1318, -18.906) (-190.3568, -18.681) (-190.3568, -18.406) knots 2 2 2 2 3 3 3 3
  line L195 (-190.3568, -18.406) -> (-190.3568, -5.4062)
  spline S196 degree 3 poles (-190.3568, -5.4062) (-190.3568, -5.1311) (-190.1318, -4.9062) (-189.8569, -4.9062) knots 4 4 4 4 5 5 5 5
  line L196 (-189.8569, -4.9062) -> (-176.8568, -4.9062)
  spline S197 degree 3 poles (-176.8568, -4.9062) (-176.5816, -4.9062) (-176.3566, -5.1311) (-176.3566, -5.4062) knots 6 6 6 6 7 7 7 7
  line L197 (-176.3566, -5.4062) -> (-176.3566, -18.406)
  spline S198 degree 3 poles (-157.3066, 24.4559) (-157.3066, 24.1808) (-157.5316, 23.9558) (-157.8068, 23.9558) knots 0 0 0 0 1 1 1 1
  line L198 (-157.8068, 23.9558) -> (-170.8069, 23.9558)
  spline S199 degree 3 poles (-170.8069, 23.9558) (-171.0818, 23.9558) (-171.3068, 24.1808) (-171.3068, 24.4559) knots 2 2 2 2 3 3 3 3
  line L199 (-171.3068, 24.4559) -> (-171.3068, 37.456)
  spline S200 degree 3 poles (-171.3068, 37.456) (-171.3068, 37.7311) (-171.0818, 37.956) (-170.8069, 37.956) knots 4 4 4 4 5 5 5 5
  line L200 (-170.8069, 37.956) -> (-157.8068, 37.956)
  spline S201 degree 3 poles (-157.8068, 37.956) (-157.5316, 37.956) (-157.3066, 37.7311) (-157.3066, 37.456) knots 6 6 6 6 7 7 7 7
  line L201 (-157.3066, 37.456) -> (-157.3066, 24.4559)
  spline S202 degree 3 poles (4.9055, 56.506) (4.9055, 56.7811) (5.1304, 57.006) (5.4054, 57.006) knots 0 0 0 0 1 1 1 1
  line L202 (5.4054, 57.006) -> (18.4054, 57.006)
  spline S203 degree 3 poles (18.4054, 57.006) (18.6807, 57.006) (18.9057, 56.7811) (18.9057, 56.506) knots 2 2 2 2 3 3 3 3
  line L203 (18.9057, 56.506) -> (18.9057, 43.5059)
  spline S204 degree 3 poles (18.9057, 43.5059) (18.9057, 43.2308) (18.6807, 43.0058) (18.4054, 43.0058) knots 4 4 4 4 5 5 5 5
  line L204 (18.4054, 43.0058) -> (5.4054, 43.0058)
  spline S205 degree 3 poles (5.4054, 43.0058) (5.1304, 43.0058) (4.9055, 43.2308) (4.9055, 43.5059) knots 6 6 6 6 7 7 7 7
  line L205 (4.9055, 43.5059) -> (4.9055, 56.506)
  spline S206 degree 3 poles (-157.3066, 0.6441) (-157.3066, 0.369) (-157.5316, 0.144) (-157.8068, 0.144) knots 0 0 0 0 1 1 1 1
  line L206 (-157.8068, 0.144) -> (-170.8069, 0.144)
  spline S207 degree 3 poles (-170.8069, 0.144) (-171.0818, 0.144) (-171.3068, 0.369) (-171.3068, 0.6441) knots 2 2 2 2 3 3 3 3
  line L207 (-171.3068, 0.6441) -> (-171.3068, 13.6438)
  spline S208 degree 3 poles (-171.3068, 13.6438) (-171.3068, 13.9189) (-171.0818, 14.1438) (-170.8069, 14.1438) knots 4 4 4 4 5 5 5 5
  line L208 (-170.8069, 14.1438) -> (-157.8068, 14.1438)
  spline S209 degree 3 poles (-157.8068, 14.1438) (-157.5316, 14.1438) (-157.3066, 13.9189) (-157.3066, 13.6438) knots 6 6 6 6 7 7 7 7
  line L209 (-157.3066, 13.6438) -> (-157.3066, 0.6441)
  spline S210 degree 3 poles (-138.2566, -56.506) (-138.2566, -56.7811) (-138.4816, -57.006) (-138.7568, -57.006) knots 0 0 0 0 1 1 1 1
  line L210 (-138.7568, -57.006) -> (-151.7569, -57.006)
  spline S211 degree 3 poles (-151.7569, -57.006) (-152.0318, -57.006) (-152.2568, -56.7811) (-152.2568, -56.506) knots 2 2 2 2 3 3 3 3
  line L211 (-152.2568, -56.506) -> (-152.2568, -43.5062)
  spline S212 degree 3 poles (-152.2568, -43.5062) (-152.2568, -43.2312) (-152.0318, -43.0062) (-151.7569, -43.0062) knots 4 4 4 4 5 5 5 5
  line L212 (-151.7569, -43.0062) -> (-138.7568, -43.0062)
  spline S213 degree 3 poles (-138.7568, -43.0062) (-138.4816, -43.0062) (-138.2566, -43.2312) (-138.2566, -43.5062) knots 6 6 6 6 7 7 7 7
  line L213 (-138.2566, -43.5062) -> (-138.2566, -56.506)
  spline S214 degree 3 poles (-138.2566, 0.6441) (-138.2566, 0.369) (-138.4816, 0.144) (-138.7568, 0.144) knots 0 0 0 0 1 1 1 1
  line L214 (-138.7568, 0.144) -> (-151.7569, 0.144)
  spline S215 degree 3 poles (-151.7569, 0.144) (-152.0318, 0.144) (-152.2568, 0.369) (-152.2568, 0.6441) knots 2 2 2 2 3 3 3 3
  line L215 (-152.2568, 0.6441) -> (-152.2568, 13.6438)
  spline S216 degree 3 poles (-152.2568, 13.6438) (-152.2568, 13.9189) (-152.0318, 14.1438) (-151.7569, 14.1438) knots 4 4 4 4 5 5 5 5
  line L216 (-151.7569, 14.1438) -> (-138.7568, 14.1438)
  spline S217 degree 3 poles (-138.7568, 14.1438) (-138.4816, 14.1438) (-138.2566, 13.9189) (-138.2566, 13.6438) knots 6 6 6 6 7 7 7 7
  line L217 (-138.2566, 13.6438) -> (-138.2566, 0.6441)
  spline S218 degree 3 poles (-71.2946, 56.506) (-71.2946, 56.7811) (-71.0696, 57.006) (-70.7947, 57.006) knots 0 0 0 0 1 1 1 1
  line L218 (-70.7947, 57.006) -> (-57.795, 57.006)
  spline S219 degree 3 poles (-57.795, 57.006) (-57.5197, 57.006) (-57.2947, 56.7811) (-57.2947, 56.506) knots 2 2 2 2 3 3 3 3
  line L219 (-57.2947, 56.506) -> (-57.2947, 43.5059)
  spline S220 degree 3 poles (-57.2947, 43.5059) (-57.2947, 43.2308) (-57.5197, 43.0058) (-57.795, 43.0058) knots 4 4 4 4 5 5 5 5
  line L220 (-57.795, 43.0058) -> (-70.7947, 43.0058)
  spline S221 degree 3 poles (-70.7947, 43.0058) (-71.0696, 43.0058) (-71.2946, 43.2308) (-71.2946, 43.5059) knots 6 6 6 6 7 7 7 7
  line L221 (-71.2946, 43.5059) -> (-71.2946, 56.506)
  spline S222 degree 3 poles (-138.2566, -37.456) (-138.2566, -37.7311) (-138.4816, -37.956) (-138.7568, -37.956) knots 0 0 0 0 1 1 1 1
  line L222 (-138.7568, -37.956) -> (-151.7569, -37.956)
  spline S223 degree 3 poles (-151.7569, -37.956) (-152.0318, -37.956) (-152.2568, -37.7311) (-152.2568, -37.456) knots 2 2 2 2 3 3 3 3
  line L223 (-152.2568, -37.456) -> (-152.2568, -24.4562)
  spline S224 degree 3 poles (-152.2568, -24.4562) (-152.2568, -24.1811) (-152.0318, -23.9562) (-151.7569, -23.9562) knots 4 4 4 4 5 5 5 5
  line L224 (-151.7569, -23.9562) -> (-138.7568, -23.9562)
  spline S225 degree 3 poles (-138.7568, -23.9562) (-138.4816, -23.9562) (-138.2566, -24.1811) (-138.2566, -24.4562) knots 6 6 6 6 7 7 7 7
  line L225 (-138.2566, -24.4562) -> (-138.2566, -37.456)
  spline S226 degree 3 poles (23.9555, 56.506) (23.9555, 56.7811) (24.1805, 57.006) (24.4554, 57.006) knots 0 0 0 0 1 1 1 1
  line L226 (24.4554, 57.006) -> (37.4554, 57.006)
  spline S227 degree 3 poles (37.4554, 57.006) (37.7307, 57.006) (37.9557, 56.7811) (37.9557, 56.506) knots 2 2 2 2 3 3 3 3
  line L227 (37.9557, 56.506) -> (37.9557, 43.5059)
  spline S228 degree 3 poles (37.9557, 43.5059) (37.9557, 43.2308) (37.7307, 43.0058) (37.4554, 43.0058) knots 4 4 4 4 5 5 5 5
  line L228 (37.4554, 43.0058) -> (24.4554, 43.0058)
  spline S229 degree 3 poles (24.4554, 43.0058) (24.1805, 43.0058) (23.9555, 43.2308) (23.9555, 43.5059) knots 6 6 6 6 7 7 7 7
  line L229 (23.9555, 43.5059) -> (23.9555, 56.506)
  spline S230 degree 3 poles (-119.2066, -56.506) (-119.2066, -56.7811) (-119.4315, -57.006) (-119.7068, -57.006) knots 0 0 0 0 1 1 1 1
  line L230 (-119.7068, -57.006) -> (-132.7069, -57.006)
  spline S231 degree 3 poles (-132.7069, -57.006) (-132.9818, -57.006) (-133.2068, -56.7811) (-133.2068, -56.506) knots 2 2 2 2 3 3 3 3
  line L231 (-133.2068, -56.506) -> (-133.2068, -43.5062)
  spline S232 degree 3 poles (-133.2068, -43.5062) (-133.2068, -43.2312) (-132.9818, -43.0062) (-132.7069, -43.0062) knots 4 4 4 4 5 5 5 5
  line L232 (-132.7069, -43.0062) -> (-119.7068, -43.0062)
  spline S233 degree 3 poles (-119.7068, -43.0062) (-119.4315, -43.0062) (-119.2066, -43.2312) (-119.2066, -43.5062) knots 6 6 6 6 7 7 7 7
  line L233 (-119.2066, -43.5062) -> (-119.2066, -56.506)
  spline S234 degree 3 poles (-138.2566, 43.5059) (-138.2566, 43.2308) (-138.4816, 43.0058) (-138.7568, 43.0058) knots 0 0 0 0 1 1 1 1
  line L234 (-138.7568, 43.0058) -> (-151.7569, 43.0058)
  spline S235 degree 3 poles (-151.7569, 43.0058) (-152.0318, 43.0058) (-152.2568, 43.2308) (-152.2568, 43.5059) knots 2 2 2 2 3 3 3 3
  line L235 (-152.2568, 43.5059) -> (-152.2568, 56.506)
  spline S236 degree 3 poles (-152.2568, 56.506) (-152.2568, 56.7811) (-152.0318, 57.006) (-151.7569, 57.006) knots 4 4 4 4 5 5 5 5
  line L236 (-151.7569, 57.006) -> (-138.7568, 57.006)
  spline S237 degree 3 poles (-138.7568, 57.006) (-138.4816, 57.006) (-138.2566, 56.7811) (-138.2566, 56.506) knots 6 6 6 6 7 7 7 7
  line L237 (-138.2566, 56.506) -> (-138.2566, 43.5059)
  spline S238 degree 3 poles (76.8436, -18.906) (76.5687, -18.906) (76.3437, -18.681) (76.3437, -18.406) knots 0 0 0 0 1 1 1 1
  line L238 (76.3437, -18.406) -> (76.3437, -5.4062)
  spline S239 degree 3 poles (76.3437, -5.4062) (76.3437, -5.1311) (76.5687, -4.9062) (76.8436, -4.9062) knots 2 2 2 2 3 3 3 3
  line L239 (76.8436, -4.9062) -> (89.8433, -4.9062)
  spline S240 degree 3 poles (89.8433, -4.9062) (90.1186, -4.9062) (90.3436, -5.1311) (90.3436, -5.4062) knots 4 4 4 4 5 5 5 5
  line L240 (90.3436, -5.4062) -> (90.3436, -18.406)
  spline S241 degree 3 poles (90.3436, -18.406) (90.3436, -18.681) (90.1186, -18.906) (89.8433, -18.906) knots 6 6 6 6 7 7 7 7
  line L241 (89.8433, -18.906) -> (76.8436, -18.906)
  spline S242 degree 3 poles (-33.1946, 32.6938) (-33.1946, 32.9689) (-32.9696, 33.1939) (-32.6947, 33.1939) knots 0 0 0 0 1 1 1 1
  line L242 (-32.6947, 33.1939) -> (-19.6946, 33.1939)
  spline S243 degree 3 poles (-19.6946, 33.1939) (-19.4193, 33.1939) (-19.1944, 32.9689) (-19.1944, 32.6938) knots 2 2 2 2 3 3 3 3
  line L243 (-19.1944, 32.6938) -> (-19.1944, 19.6941)
  spline S244 degree 3 poles (-19.1944, 19.6941) (-19.1944, 19.419) (-19.4193, 19.194) (-19.6946, 19.194) knots 4 4 4 4 5 5 5 5
  line L244 (-19.6946, 19.194) -> (-32.6947, 19.194)
  spline S245 degree 3 poles (-32.6947, 19.194) (-32.9696, 19.194) (-33.1946, 19.419) (-33.1946, 19.6941) knots 6 6 6 6 7 7 7 7
  line L245 (-33.1946, 19.6941) -> (-33.1946, 32.6938)
  spline S246 degree 3 poles (-157.3066, -37.456) (-157.3066, -37.7311) (-157.5316, -37.956) (-157.8068, -37.956) knots 0 0 0 0 1 1 1 1
  line L246 (-157.8068, -37.956) -> (-170.8069, -37.956)
  spline S247 degree 3 poles (-170.8069, -37.956) (-171.0818, -37.956) (-171.3068, -37.7311) (-171.3068, -37.456) knots 2 2 2 2 3 3 3 3
  line L247 (-171.3068, -37.456) -> (-171.3068, -24.4562)
  spline S248 degree 3 poles (-171.3068, -24.4562) (-171.3068, -24.1811) (-171.0818, -23.9562) (-170.8069, -23.9562) knots 4 4 4 4 5 5 5 5
  line L248 (-170.8069, -23.9562) -> (-157.8068, -23.9562)
  spline S249 degree 3 poles (-157.8068, -23.9562) (-157.5316, -23.9562) (-157.3066, -24.1811) (-157.3066, -24.4562) knots 6 6 6 6 7 7 7 7
  line L249 (-157.3066, -24.4562) -> (-157.3066, -37.456)
  spline S250 degree 3 poles (-119.2066, 24.4559) (-119.2066, 24.1808) (-119.4315, 23.9558) (-119.7068, 23.9558) knots 0 0 0 0 1 1 1 1
  line L250 (-119.7068, 23.9558) -> (-132.7069, 23.9558)
  spline S251 degree 3 poles (-132.7069, 23.9558) (-132.9818, 23.9558) (-133.2068, 24.1808) (-133.2068, 24.4559) knots 2 2 2 2 3 3 3 3
  line L251 (-133.2068, 24.4559) -> (-133.2068, 37.456)
  spline S252 degree 3 poles (-133.2068, 37.456) (-133.2068, 37.7311) (-132.9818, 37.956) (-132.7069, 37.956) knots 4 4 4 4 5 5 5 5
  line L252 (-132.7069, 37.956) -> (-119.7068, 37.956)
  spline S253 degree 3 poles (-119.7068, 37.956) (-119.4315, 37.956) (-119.2066, 37.7311) (-119.2066, 37.456) knots 6 6 6 6 7 7 7 7
  line L253 (-119.2066, 37.456) -> (-119.2066, 24.4559)
  spline S254 degree 3 poles (-176.3566, -56.506) (-176.3566, -56.7811) (-176.5816, -57.006) (-176.8568, -57.006) knots 0 0 0 0 1 1 1 1
  line L254 (-176.8568, -57.006) -> (-189.8569, -57.006)
  spline S255 degree 3 poles (-189.8569, -57.006) (-190.1318, -57.006) (-190.3568, -56.7811) (-190.3568, -56.506) knots 2 2 2 2 3 3 3 3
  line L255 (-190.3568, -56.506) -> (-190.3568, -43.5062)
  spline S256 degree 3 poles (-190.3568, -43.5062) (-190.3568, -43.2312) (-190.1318, -43.0062) (-189.8569, -43.0062) knots 4 4 4 4 5 5 5 5
  line L256 (-189.8569, -43.0062) -> (-176.8568, -43.0062)
  spline S257 degree 3 poles (-176.8568, -43.0062) (-176.5816, -43.0062) (-176.3566, -43.2312) (-176.3566, -43.5062) knots 6 6 6 6 7 7 7 7
  line L257 (-176.3566, -43.5062) -> (-176.3566, -56.506)
  spline S258 degree 3 poles (-119.2066, -37.456) (-119.2066, -37.7311) (-119.4315, -37.956) (-119.7068, -37.956) knots 0 0 0 0 1 1 1 1
  line L258 (-119.7068, -37.956) -> (-132.7069, -37.956)
  spline S259 degree 3 poles (-132.7069, -37.956) (-132.9818, -37.956) (-133.2068, -37.7311) (-133.2068, -37.456) knots 2 2 2 2 3 3 3 3
  line L259 (-133.2068, -37.456) -> (-133.2068, -24.4562)
  spline S260 degree 3 poles (-133.2068, -24.4562) (-133.2068, -24.1811) (-132.9818, -23.9562) (-132.7069, -23.9562) knots 4 4 4 4 5 5 5 5
  line L260 (-132.7069, -23.9562) -> (-119.7068, -23.9562)
  spline S261 degree 3 poles (-119.7068, -23.9562) (-119.4315, -23.9562) (-119.2066, -24.1811) (-119.2066, -24.4562) knots 6 6 6 6 7 7 7 7
  line L261 (-119.2066, -24.4562) -> (-119.2066, -37.456)
  spline S262 degree 3 poles (47.7687, -24.4562) (47.7687, -24.1811) (47.9937, -23.9562) (48.2686, -23.9562) knots 0 0 0 0 1 1 1 1
  line L262 (48.2686, -23.9562) -> (61.2673, -23.9562)
  spline S263 degree 3 poles (61.2673, -23.9562) (61.5425, -23.9562) (61.7675, -24.1811) (61.7675, -24.4562) knots 2 2 2 2 3 3 3 3
  line L263 (61.7675, -24.4562) -> (61.7675, -37.456)
  spline S264 degree 3 poles (61.7675, -37.456) (61.7675, -37.7311) (61.5425, -37.956) (61.2673, -37.956) knots 4 4 4 4 5 5 5 5